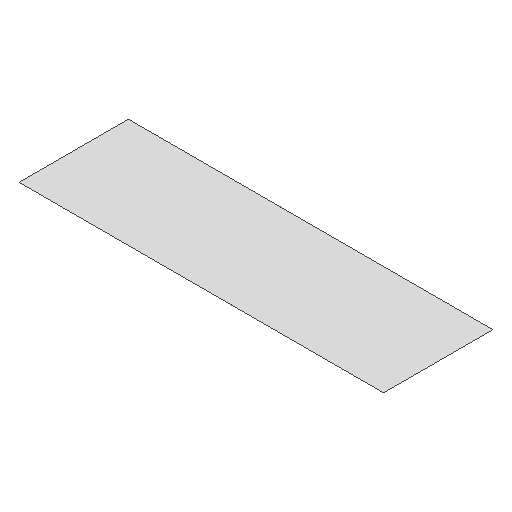
# Autodesk Inventor part: Loop plane
Saved by Autodesk Inventor 2026.1 (Build 301233000, 233)
## iProperties
Created: 2025-08-15
Part Number: Loop plane
Material: Generic
Document SubType Name: Modeling
Designer: farin012
Density: 1 g/cm^3
Appearance: Default
Author: farin012
Autodesk Inventor part; units mm, degrees
ref_plane "YZ Plane" through (0, 0, 0) normal (1, 0, 0) x (0, 1, 0)
ref_plane "XZ Plane" through (0, 0, 0) normal (0, 1, 0) x (-1, 0, 0)
ref_plane "XY Plane" through (0, 0, 0) normal (0, 0, 1) x (1, 0, 0)
sketch "Sketch1" plane through (0, 0, 0) normal (0, 1, 0) x (-1, 0, 0)
  line L0 (127, 38.1) -> (-127, 38.1)
  line L1 (-127, 38.1) -> (-127, -38.1)
  line L2 (-127, -38.1) -> (127, -38.1)
  line L3 (127, -38.1) -> (127, 38.1)
  line L4 (127, 38.1) -> (-127, -38.1) construction
  line L5 (-127, 38.1) -> (127, -38.1) construction
  point P0 (0, 0)
  dimension "d0" = 254
  dimension "d1" = 76.2
  constraints: 12 end point, 2 midpoint, 2 parallel, 1 horizontal, 1 perpendicular
  measures "d0" distance of L2.end L1.end
  measures "d1" distance of L1.end L0.end
extrude "Extrusion1" add sketch "Sketch1" along normal blind 0.0005
body "Solid1"
